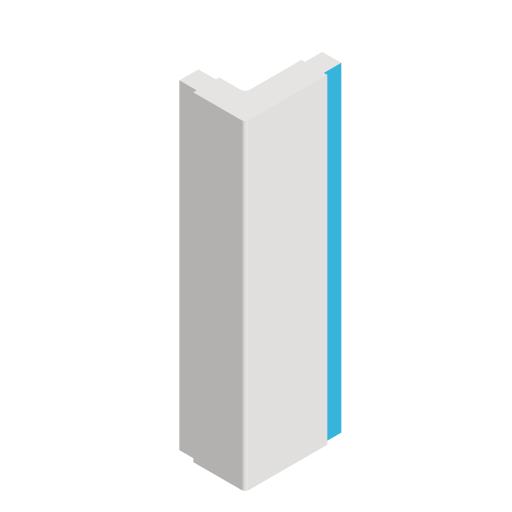
# Autodesk Inventor part: Столбик
Saved by Autodesk Inventor 2023.2 (Build 272271030, 271C)
## iProperties
Created: 2025-04-23
Part Number: Столбик
Material: Типовые
Document SubType Name: Modeling
Designer: Коноваленко
Density: 1 g/cm^3
Appearance: По умолчанию
Author: Коноваленко
Autodesk Inventor part; units mm, degrees
ref_plane "YZ Plane" through (0, 0, 0) normal (1, 0, 0) x (0, 1, 0)
ref_plane "XZ Plane" through (0, 0, 0) normal (0, 1, 0) x (-1, 0, 0)
ref_plane "XY Plane" through (0, 0, 0) normal (0, 0, 1) x (1, 0, 0)
sketch "Эскиз1" plane through (0, 0, 0) normal (0, 1, 0) x (-1, 0, 0)
  line L0 (-30, -85) -> (-30, 30)
  line L1 (-30, 30) -> (50, 30)
  line L2 (50, 30) -> (50, 0)
  line L3 (50, 0) -> (0, 0)
  line L4 (0, 0) -> (0, -85)
  line L5 (0, -85) -> (-30, -85)
  circle A0 centre (-26, 26) radius 4
  line L6 (50, 26) -> (30, 26)
  line L7 (30, 26) -> (30, 30)
  circle A1 centre (5, -5) radius 5
  line L8 (-30, -85) -> (-26, -85)
  line L9 (-26, -85) -> (-26, -65)
  line L10 (-26, -65) -> (-30, -65)
  line L11 (-30, -65) -> (-30, -85)
  line L12 (0, -85) -> (-4, -85)
  line L13 (-4, -85) -> (-4, -65)
  line L14 (-4, -65) -> (0, -65)
  line L15 (0, -65) -> (0, -85)
  line L16 (50, 0) -> (30, 0)
  line L17 (30, 0) -> (30, 4)
  line L18 (30, 4) -> (50, 4)
  line L19 (50, 4) -> (50, 0)
  point P0 (-26, 30)
  point P1 (-30, 26)
  point P2 (0, -5)
  point P3 (5, 0)
  point P4 (50, 4)
  point P5 (0, -65)
  point P6 (30, 0)
  dimension "d0" = 80
  dimension "d1" = 115
  dimension "d2" = 30
  dimension "d3" = 30
  dimension "d6" = 4
  dimension "d7" = 20
  dimension "d8" = 10
  dimension "d9" = 4
  dimension "d10" = 20
  dimension "d26" = 8
  dimension "d27" = 4
  dimension "d28" = 20
  dimension "d29" = 4
  dimension "d30" = 20
  constraints: 40 end point, 9 perpendicular, 6 parallel, 4 horizontal, 4 point on line, 4 tangent, 2 centre point, 1 vertical
  measures "d0" distance of L0.end L1.end
  measures "d1" distance of L0.start L0.end
  measures "d2" distance between parallel lines of L1 L3
  measures "d3" distance between parallel lines of L0 L4
  measures "d6" distance between parallel lines of L6 L1
  measures "d7" distance between parallel lines of L2 L7
  measures "d8" diameter of A1
  measures "d9" distance between parallel lines of L0 L9
  measures "d10" distance of L8.end L9.end
  measures "d26" diameter of A0
  measures "d27" distance of L13.end L14.end
  measures "d28" distance of L12.end L13.end
  measures "d29" distance between parallel lines of L3 L18
  measures "d30" distance of L17.end L18.end
extrude "Выдавливание1" add sketch "Эскиз1" along normal blind 370 contours L0 A0 L1 L7 L6 L2 L18 L17 L3 L4 L14 L13 L5 L9 L10 | A0 | L4 L3 A1
sketch "Эскиз2" plane through (0, 0, 0) normal (0, -1, 0) x (1, 0, 0)
  line L0 (-5, 0) -> (-30, 0) projected
  line L1 (-20, 0) -> (-20, 10)
  line L2 (-20, 10) -> (10, 10)
  line L3 (10, 10) -> (10, -35)
  line L4 (10, -35) -> (0, -35)
  line L5 (0, -65) -> (0, -5) projected
  arc A0 (0, -5) -> (-5, 0) centre (-5, -5) ccw projected
  line L6 (0, -65) -> (0, -5) projected
  point P0 (0, 0)
  point P1 (-60, 0)
  point P2 (0, -60)
  point P3 (-20, 5)
  dimension "d15" = 10
  dimension "d16" = 10
  dimension "d17" = 30
  constraints: 8 end point, 4 perpendicular, 2 midpoint, 1 point on line
  measures "d15" distance between parallel lines of L0 L2
  measures "d16" distance between parallel lines of L5 L3
  measures "d17" distance from line of point (-20, 5) L3
extrude "Выдавливание2" cut sketch "Эскиз2" against normal blind 100
extrude "Выдавливание3" add sketch "Эскиз2" against normal blind 40
fillet "Сопряжение1" radius 2 15 edges at (-5, 100, 10) (10, 100, -12.5) (10, 70, 10) (10, 40, -12.5) (-5, 40, 10) (10, 70, -35) (-20, 70, 10) (-1.4645, 100, -1.4645) (-12.5, 100, 0) (0, 100, -20) (-1.4645, 40, -1.4645) (0, 40, -20) (-12.5, 40, 0) (0, 70, -35) (-20, 70, 0)
sketch "Эскиз13" plane through (0, 370, 0) normal (0, 1, 0) x (1, 0, 0)
  line L0 (4, 85) -> (4, 65) projected
  line L1 (26, 65) -> (26, 85) projected
  line L2 (26, 85) -> (4, 85) projected
  line L3 (4, 65) -> (0, 65) projected
  line L4 (30, 65) -> (26, 65) projected
  line L5 (0, 65) -> (0, 5) projected
  line L6 (0, 32.67) -> (30, 32.67)
  line L7 (30, -26) -> (30, 65) projected
  point P0 (0, 0)
  dimension "d130" = 52.33
  constraints: 2 end point, 2 point on line, 1 horizontal
  measures "d130" distance between parallel lines of L2 L6
extrude "Выдавливание11" [suppressed]
mirror "Зеркальное отражение5" [suppressed]
